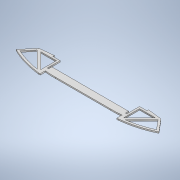
# Autodesk Inventor part: bulkhead_front
Saved by Autodesk Inventor 2020.3 (Build 243373000, 373)
## iProperties
Created: 2020-05-22
Part Number: bulkhead_front
Material: Generic
Document SubType Name: Modeling
Designer: kardo
Density: 1 g/cm^3
Appearance: Default
Mass: 5.03512 g
Surface Area: 68.3965 cm^2
Volume: 5.03512 cm^3
Author: kardo
Autodesk Inventor part; units mm, degrees
ref_plane "YZ Plane" through (0, 0, 0) normal (1, 0, 0) x (0, 1, 0)
ref_plane "XZ Plane" through (0, 0, 0) normal (0, 1, 0) x (-1, 0, 0)
ref_plane "XY Plane" through (0, 0, 0) normal (0, 0, 1) x (1, 0, 0)
derived "base_sketch.ipt"
sketch "bulkhead_front" plane through (0, 112.2, 32.9472) normal (0, 1, 0) x (-1, 0, 0)
  line L0 (-33.539, -25.2071) -> (-11.5056, -27.5882)
  line L1 (-11.5056, -27.5882) -> (-11.5056, -25.1014)
  line L2 (-11.5056, -25.1014) -> (0, -25.1014)
  line L3 (19.176, 13.8708) -> (62.322, 13.8708)
  line L4 (-11.5056, -35.434) -> (-34.5168, -32.9472)
  line L5 (-11.5056, -32.9472) -> (-11.5056, -35.434)
  line L6 (0, -32.9472) -> (-11.5056, -32.9472)
  line L7 (-34.5168, -32.9472) -> (-57.528, -5.4072)
  line L8 (0, -13.2972) -> (28.764, -13.2972)
  line L9 (28.764, -19.7029) -> (62.322, -19.7029)
  line L10 (28.764, -13.2972) -> (28.764, -19.7029)
  line L11 (62.322, 13.8708) -> (62.322, -19.7029)
  line L12 (0, -13.2972) -> (0, -32.9472)
  line L13 (0, -25.1014) -> (0, -10.0406)
  line L14 (0, -10.0406) -> (62.322, -10.0406)
  line L15 (19.176, 0.918) -> (62.322, 0.918)
  line L16 (-38.352, -0.8129) -> (-38.352, 3.7728) construction
  line L17 (-19.176, 5.0623) -> (-19.176, 9.648) construction
  line L18 (0, 8.3671) -> (0, 12.9528) construction
  line L19 (-57.528, -5.4072) -> (-57.528, -9.9929) construction
  line L20 (-33.539, -25.2071) -> (-49.746, -5.8104)
  line L21 (0, 8.3671) -> (0, 0)
  line L22 (-57.528, -7.15) -> (0, 2.7528) construction
  spline S0 degree 4 poles (-57.528, -5.4072) (-46.0483, 1.2579) (-30.6129, 7.5809) (-11.2214, 12.0942) (8.3201, 13.8708) (15.5662, 13.8708) (19.176, 13.8708) knots 0 0 0 0 0 0.630279 0.815816 1 1 1 1 1
  spline S1 degree 3 poles (-57.528, -9.9929) (-39.18, 0.6762) (-19.6272, 6.1032) (0, 8.3671) knots 0 0 0 0 1 1 1 1
  spline S2 degree 3 poles (0, 0) (6.37, 0.918) (12.773, 0.918) (19.176, 0.918) knots 0 0 0 0 1 1 1 1
ref_plane "bulkhead_front_plane" through (0, 112.2, 32.9472) normal (0, 1, 0) x (-1, 0, 0)
sketch "Sketch2" plane through (0, 112.2, 32.9472) normal (0, 1, 0) x (-1, 0, 0)
  spline S0 degree 3 poles (-57.528, -9.9929) (-39.18, 0.6762) (-19.6272, 6.1032) (0, 8.3671) knots 0 0 0 0 1 1 1 1 projected
  line L0 (-33.539, -25.2071) -> (-49.746, -5.8104) projected
  line L1 (-33.539, -25.2071) -> (-11.5056, -27.5882) projected
  line L2 (-11.5056, -25.1014) -> (0, -25.1014) projected
  line L3 (-11.5056, -27.5882) -> (-11.5056, -25.1014) projected
  line L4 (0, -25.1014) -> (0, -10.0406) projected
  line L5 (0, -10.0406) -> (62.322, -10.0406) projected
  spline S1 degree 3 poles (0, 0) (6.37, 0.918) (12.773, 0.918) (19.176, 0.918) knots 0 0 0 0 1 1 1 1 projected
  line L6 (19.176, 0.918) -> (62.322, 0.918) projected
  line L7 (0, 8.3671) -> (0, 0) projected
  line L8 (62.322, 13.8708) -> (62.322, -19.7029) projected
  line L9 (-44.9651, -6.8535) -> (-32.6978, -21.5351)
  line L10 (-33.539, -25.2071) -> (0, 8.3671) construction
  line L11 (-3, 2.5341) -> (-3, -22.1014)
  line L12 (-3, -22.1014) -> (-27.6097, -22.1014)
  line L13 (-27.6097, -22.1014) -> (-3, 2.5341)
  line L14 (-32.6978, -21.5351) -> (-6.7689, 4.421)
  spline S2 degree 2 poles (-44.9651, -6.8535) (-26.6462, 1.4235) (-6.7689, 4.421) knots 0 0 0 1 1 1
  line L15 (-44.9651, -6.8535) -> (-46.2168, -4.1271) construction
  line L16 (-26.2566, 0.1036) -> (-27.0971, 2.9835) construction
  line L17 (-6.7689, 4.421) -> (-7.2338, 7.3848) construction
  line L18 (-44.9651, -6.8535) -> (-26.2566, 0.1036) construction
  line L19 (-6.7689, 4.421) -> (-26.2566, 0.1036) construction
  line L20 (0, 8.3671) -> (2, 8.3671)
  line L21 (2, 8.3671) -> (2, 0.259)
  line L22 (0, -10.0406) -> (0, -5.0203)
  line L23 (0, -5.0203) -> (2, -5.0203)
  line L24 (2, -5.0203) -> (2, -10.0406)
  line L25 (0, -5.0203) -> (0, 0) construction
  point P0 (0, -32.9472)
  dimension "d1" = 3
  dimension "d2" = 3
  dimension "d3" = 3
  dimension "d4" = 4
  dimension "d5" = 3
  dimension "d6" = 2
  constraints: 34 end point, 4 equal length, 4 parallel, 3 vertical, 2 perpendicular, 1 collinear, 1 horizontal, 1 point on line, 11 other
  measures "d1" distance between parallel lines of L2 L12
  measures "d2" distance between parallel lines of L4 L11
  measures "d3" distance of L9.start L15.end
  measures "d4" distance between parallel lines of L13 L14
  measures "d5" distance between parallel lines of L0 L9
  measures "d6" distance between parallel lines of L24 L22
extrude "Extrusion1" add sketch "Sketch2" along normal blind 2 contours S0 L7 S1 L6 L8 L5 L24 L23 L22 L4 L2 L3 L1 L0 | L20 L21 S1 L7
mirror "Mirror1" about plane through (-62.322, 112.2, 22.9066) normal (-1, 0, 0) of "Extrusion1"
equation "\"d6\" = stringer_thickness"
equation "\"d7\" = bulkhead_thickness"
equation "\"stringer_thickness\" = 2"
equation "\"bulkhead_thickness\" = 2"
body "Solid1"
